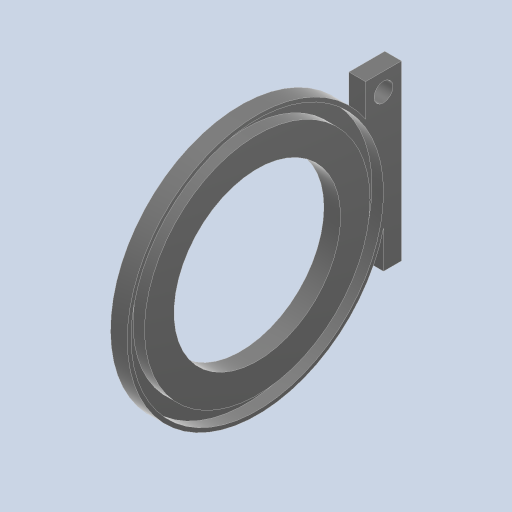
# Autodesk Inventor part: RFID_holder_coil_01
Saved by Autodesk Inventor 2024.4 (Build 284460000, 460)
## iProperties
Created: 2026-03-24
Part Number: RFID_holder_coil_01
Material: PLA Black
Document SubType Name: Modeling
Designer: Admin
Density: 1.06 g/cm^3
Appearance: Smooth - White(2)
Author: Admin
Autodesk Inventor part; units mm, degrees
note: some values were not read from the file. Chosen so that the rebuilt part matches the saved one: second side of "Ex2: RFID holder base".
ref_plane "YZ Plane" through (0, 0, 0) normal (1, 0, 0) x (0, 1, 0)
ref_plane "XZ Plane" through (0, 0, 0) normal (0, 1, 0) x (-1, 0, 0)
ref_plane "XY Plane" through (0, 0, 0) normal (0, 0, 1) x (1, 0, 0)
sketch "Sketch2: RFID holder" plane through (0, 0, 0) normal (1, 0, 0) x (0, 0, -1)
  circle A0 centre (-28.125, 0) radius 16.25
  circle A1 centre (-28.125, 0) radius 22
  circle A2 centre (-28.125, 0) radius 24.625
  circle A3 centre (-28.125, 0) radius 25.375
  line L0 (-28.125, 1.5) -> (0, 1.5)
  line L1 (-28.125, -1.5) -> (0, -1.5)
  line L2 (0, -13.4) -> (0, 13.4)
  line L3 (0, -13.4) -> (-3.5, -13.4)
  line L4 (0, 13.4) -> (-3.5, 13.4)
  line L5 (-3.5, 13.4) -> (-3.5, -13.4)
  line L6 (-28.125, 1.5) -> (-28.125, -1.5) construction
  line L7 (-2.75, 13.4) -> (-2.75, -13.4) construction
  line L8 (-1, 13.4) -> (-1, -13.4)
  line L9 (-3.5, -6.1237) -> (0, -6.1237)
  point P0 (-2.7944, -1.5)
  point P1 (-2.7944, 1.5)
  point P2 (0, 0)
  point P3 (-6.1762, -1.5)
  point P4 (-6.1762, 1.5)
  point P5 (-3.5457, -1.5)
  point P6 (-3.5457, 1.5)
  point P7 (-3.5, -1.5)
  point P8 (-3.5, 1.5)
  point P9 (-3.5, 0)
  point P10 (0, 0)
  point P11 (-3.5, 6.1237)
  point P12 (-3.5, -6.1237)
  point P13 (-1, -1.5)
  point P14 (-1, 1.5)
  dimension "d48" = 50.75
  dimension "RFID_coil_ID" = 44
  dimension "RFID_coil_OD" = 49.25
  dimension "d7" = 0.75
  dimension "d49" = 3
  dimension "d54" = 1.5
  dimension "d57" = 0.75
  dimension "d58" = 26.8
  dimension "d59" = 3.5
  dimension "d60" = 32.5
  dimension "dist_for_RFID_wire" = 2.5
  constraints: 20 end point, 8 point on line, 6 coincident, 5 perpendicular, 3 centre point, 3 midpoint, 2 horizontal, 2 horizontal alignment, 1 parallel, 1 vertical, 3 other
  measures "RFID_coil_ID" diameter of A1
  measures "RFID_coil_OD" diameter of A2
  measures "d49" distance between parallel lines of L1 L0
  measures "d54" distance of L0.start point (-28.125, 0)
  measures "d57" distance between parallel lines of L7 L5
  measures "d58" distance of L2.start L2.end
  measures "d59" distance between parallel lines of L2 L5
  measures "d60" diameter of A0
  measures "dist_for_RFID_wire" distance from line of L8 point (-3.5, 0)
sketch "Sketch8: M3 through hole" plane through (0, 0, 0) normal (1, 0, 0) x (0, 1, 0)
  line L0 (20.4, 7) -> (13.4, 7)
  line L1 (13.4, 7) -> (13.4, 0)
  line L2 (13.4, 0) -> (20.4, 0)
  line L3 (20.4, 0) -> (20.4, 7)
  circle A0 centre (16.9, 3.5) radius 1.85
  circle A1 centre (0, 28.125) radius 25.375 projected
  line L4 (13.4, 3.5) -> (-13.4, 3.5) projected
  line L5 (13.4, 0) -> (13.4, 3.5) construction
  point P0 (0, 0)
  point P1 (20.4, 3.5)
  point P2 (16.9, 7)
  point P3 (6.1237, 3.5)
  point P4 (14.0579, 7)
  dimension "d63" = 3.7
  dimension "d66" = 7
  dimension "d67" = 7
  constraints: 8 end point, 3 perpendicular, 2 midpoint, 1 centre point, 1 collinear, 1 horizontal, 1 horizontal alignment, 1 vertical alignment
  measures "d63" diameter of A0
  measures "d66" distance of L2.end L0.start
  measures "d67" distance of L1.end L2.end
extrude "Ex2: RFID holder base" add sketch "Sketch2: RFID holder" against normal blind 3.25 contours A0 L0 A1 L1 | A0 L1 A1 L0 | L0 A2 L1 A1 | A1 L1 A2 L0 | L0 L5 A2 | A2 L1 L5 A3 L0 | A2 L5 L1 | L5 L0 A3 L1 | L5 A3 L0 | L1 A3 L5 | L0 L8 L1 A3 | A3 L5 L4 L8 L0 | L1 L8 L9 A3 | L9 L8 L3 L5 | L8 L4 L2 L0 | L0 L2 L1 L8 | L1 L2 L9 L8 | L9 L2 L3 L8
extrude "Ex3: RFID inset" cut sketch "Sketch2: RFID holder" against normal blind 2.25 contours L0 A2 L1 A1 | A1 L1 A2 L0
extrude "Ex4: RFID wire cutout" [suppressed]
extrude "Ex: M3 through hole" add sketch "Sketch8: M3 through hole" against normal up to surface (3.25 mm away) contours L3 L2 L1 A1 L0 | L1 L4 A1
equation "\"d54\" = 0.5 * d49"
body "Solid1"
